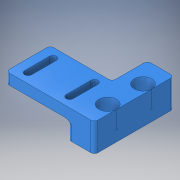
# Autodesk Inventor part: Belt_Clamp_L
Saved by Autodesk Inventor 2019.4 (Build 234330000, 330)
## iProperties
Created: 2021-02-03
Part Number: Belt_Clamp_L
Material: Generic
Document SubType Name: Modeling
Designer: Jorian Brusind
Density: 1 g/cm^3
Appearance: Cyan
Author: Jorian Brusind
Autodesk Inventor part; units mm, degrees
ref_plane "YZ Plane" through (0, 0, 0) normal (1, 0, 0) x (0, 1, 0)
ref_plane "XZ Plane" through (0, 0, 0) normal (0, 1, 0) x (-1, 0, 0)
ref_plane "XY Plane" through (0, 0, 0) normal (0, 0, 1) x (1, 0, 0)
sketch "Sketch1" plane through (0, 0, 0) normal (0, 1, 0) x (-1, 0, 0)
  line L0 (0, 0) -> (50, 0)
  line L1 (50, 0) -> (50, -45)
  line L2 (50, -45) -> (0, -45)
  line L3 (0, -45) -> (0, 0)
  line L4 (50, 0) -> (50, -25)
  line L5 (50, -25) -> (15, -25)
  line L6 (15, -25) -> (15, -45)
  dimension "d0" = 50
  dimension "d1" = 45
  dimension "d13" = 25
  dimension "d14" = 35
  constraints: 14 end point, 3 perpendicular, 2 parallel, 2 point on line, 1 horizontal
  measures "d0" distance of L1.end L2.end
  measures "d1" distance of L0.end L1.end
  measures "d13" distance of L0.end L4.end
  measures "d14" distance of L4.end L5.end
extrude "Extrusion3" add sketch "Sketch1" along normal blind 6 contours L0 L1 L5 L6 L2 L3
sketch "Sketch4" plane through (0, 6, 0) normal (0, 1, 0) x (1, 0, 0)
  line L0 (-43, 5.5) -> (-43, 19.5) construction
  line L1 (-41, 5.5) -> (-41, 19.5)
  line L2 (-45, 19.5) -> (-45, 5.5)
  arc A0 (-45, 5.5) -> (-41, 5.5) centre (-43, 5.5) ccw
  arc A1 (-41, 19.5) -> (-45, 19.5) centre (-43, 19.5) ccw
  line L3 (-50, 25) -> (-50, 0) projected
  line L4 (-15, 25) -> (-50, 25) projected
  line L5 (-19.5, 19.5) -> (-19.5, 5.5) construction
  line L6 (-21.5, 19.5) -> (-21.5, 5.5)
  line L7 (-17.5, 5.5) -> (-17.5, 19.5)
  arc A2 (-17.5, 19.5) -> (-21.5, 19.5) centre (-19.5, 19.5) ccw
  arc A3 (-21.5, 5.5) -> (-17.5, 5.5) centre (-19.5, 5.5) ccw
  line L8 (-19.5, 12.5) -> (-5.5, 12.5) construction
  line L9 (-50, 0) -> (0, 0) projected
  point P0 (-43, 12.5)
  dimension "d17" = 7
  dimension "d18" = 4
  dimension "d19" = 5
  dimension "d20" = 5.5
  dimension "d21" = 7
  dimension "d22" = 90
  dimension "d23" = 4
  dimension "d25" = 19.5
  dimension "d28" = 5.5
  constraints: 18 end point, 8 point on circle, 8 tangent, 4 centre point, 2 midpoint, 2 parallel, 2 perpendicular, 1 horizontal, 1 vertical
  measures "d17" distance of point (-43, 12.5) L0.end
  measures "d18" diameter of A1
  measures "d19" distance between parallel lines of L3 L2
  measures "d20" distance from line of L4 L0.end
  measures "d21" distance of L8.start L5.end
  measures "d22" angle of L5 L8
  measures "d23" diameter of A3
  measures "d25" distance between parallel lines of L1 L6
  measures "d28" distance from line of L4 L5.start
extrude "Extrusion4" cut sketch "Sketch4" against normal up to next
sketch "Sketch7" plane through (0, 0, 0) normal (0, -1, 0) x (1, 0, 0)
  line L0 (0, 0) -> (0, -45) projected
  line L1 (0, -45) -> (-15, -45)
  line L2 (-15, -45) -> (-15, 0)
  line L3 (-15, 0) -> (0, 0)
  line L4 (0, 0) -> (0, -45)
  dimension "d38" = 15
  dimension "d39" = 45
  constraints: 8 end point, 2 parallel, 1 horizontal, 1 perpendicular
  measures "d38" distance of L2.end L3.end
  measures "d39" distance of L1.end L2.end
extrude "Extrusion6" add sketch "Sketch7" along normal blind 10
sketch "Sketch5" plane through (0, 6, 0) normal (0, 1, 0) x (1, 0, 0)
  circle A0 centre (-5, 12.5) radius 2.5
  circle A1 centre (-5, 32.5) radius 2.5
  line L0 (-50, 0) -> (0, 0) projected
  line L1 (0, 0) -> (0, 45) projected
  dimension "d29" = 5
  dimension "d30" = 5
  dimension "d31" = 12.5
  dimension "d32" = 5
  dimension "d33" = 5
  dimension "d34" = 20
  constraints: 2 centre point
  measures "d29" diameter of A0
  measures "d30" diameter of A1
  measures "d31" distance from line of L0 A0.centre
  measures "d32" distance from line of L1 A0.centre
  measures "d33" distance from line of L1 A1.centre
  measures "d34" distance of A0.centre A1.centre
extrude "Extrusion5" cut sketch "Sketch5" against normal up to next
sketch "Sketch8" plane through (0, 6, 0) normal (0, 1, 0) x (1, 0, 0)
  circle A0 centre (-5, 12.5) radius 2.5 projected
  circle A1 centre (-5, 12.5) radius 5
  circle A2 centre (-5, 32.5) radius 2.5 projected
  circle A3 centre (-5, 32.5) radius 5
  point P0 (0, 0)
  dimension "d42" = 10
  dimension "d43" = 10
  constraints: 2 centre point, 2 coincident
  measures "d42" diameter of A1
  measures "d43" diameter of A3
extrude "Extrusion7" cut sketch "Sketch8" against normal blind 10
fillet "Fillet2" radius 2 6 edges at (0, -2, 0) (0, -2, -45) (-15, -2, -45) (-15, 3, -25) (-15, -5, 0) (-15, 0, -12.5)
fillet "Fillet3" radius 2 2 edges at (-50, 3, -25) (-50, 3, 0)
body "Solid2"
